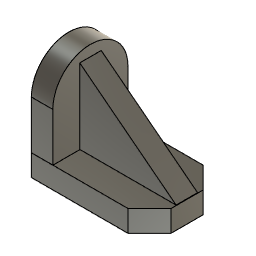
Lab#3.2 (Autodesk Fusion 360 design; units mm, degrees)
Autodesk Fusion 360 part; units mm, degrees
sketch "Horizontal" plane through (0, 0, 0) normal (0, 0, 1) x (1, 0, 0)
  line L0 (33, -21) -> (-33, -21)
  line L1 (-33, -21) -> (-33, 21)
  line L2 (-33, 21) -> (33, 21)
  line L3 (33, 21) -> (33, -21)
  line L4 (33, -21) -> (-33, 21) construction
  line L5 (-33, -21) -> (33, 21) construction
  dimension "d1" = 66
  dimension "d2" = 42
  constraint horizontal L0
  constraint perpendicular L0 L1
  constraint parallel L0 L2
  constraint parallel L1 L3
  constraint coincident L4 origin
  constraint coincident L5 origin
  measures "d1" distance of L1.end L2.end
  measures "d2" distance of L0.end L1.end
extrude "Extrude1" add sketch "Horizontal" along normal blind 12
chamfer "Chamfer1" distance 12 angle 45 2 edges at (33, -21, 6) (33, 21, 6)
sketch "Vertical" plane through (0, 0, 0) normal (0, 0, 1) x (1, 0, 0)
  line L0 (-33, 20.9715) -> (-21, 20.9715)
  line L1 (-21, 20.9715) -> (-21, -21.0285)
  line L2 (-21, -21.0285) -> (-33, -21.0285)
  line L3 (-33, -21.0285) -> (-33, 20.9715)
  line L4 (-33, 20.9715) -> (-21, 20.9715)
  line L5 (-21, 20.9715) -> (-21, -21.0285)
  line L6 (-21, -21.0285) -> (-33, -21.0285)
  line L7 (-33, -21.0285) -> (-33, 20.9715)
  line L8 (-33, -21) -> (-33, 21)
  dimension "d6" = 12
  dimension "d7" = 42
  dimension "d8" = 12
  dimension "d9" = 42
  constraint horizontal L0
  constraint vertical L1
  constraint horizontal L2
  constraint vertical L3
  constraint horizontal L4
  constraint vertical L5
  constraint horizontal L6
  constraint vertical L7
  constraint collinear L7 L8
  constraint collinear L3 L8
  constraint collinear L0 L4
  measures "d6" distance of L0.start L0.end
  measures "d7" distance of L0.start L2.end
  measures "d8" distance of L0.start L0.end
  measures "d9" distance of L0.start L2.end
extrude "Extrude2" add sketch "Vertical" along normal blind 60 and the other way blind -12
fillet "Fillet1" radius 21 2 edges at (-27, -21.0285, 60) (-27, 20.9715, 60)
sketch "Triangle" plane through (0, 0, 0) normal (0, 1, 0) x (1, 0, 0)
  line L0 (-21.1404, -54.1172) -> (-21.1404, -12.1172)
  line L1 (-21.1404, -12.1172) -> (32.8596, -12.1172)
  line L2 (32.8596, -12.1172) -> (-21.1404, -54.1172)
  dimension "d16" = 42
  dimension "d17" = 54
  constraint vertical L0
  constraint perpendicular L0 L1
  measures "d16" distance of L0.start L0.end
  measures "d17" distance of L0.end L1.end
extrude "Extrude3" add sketch "Triangle" along normal mid plane 12
equation "d17 = 66 mm - 12 mm"
named bodies: "Lab#3.2"
